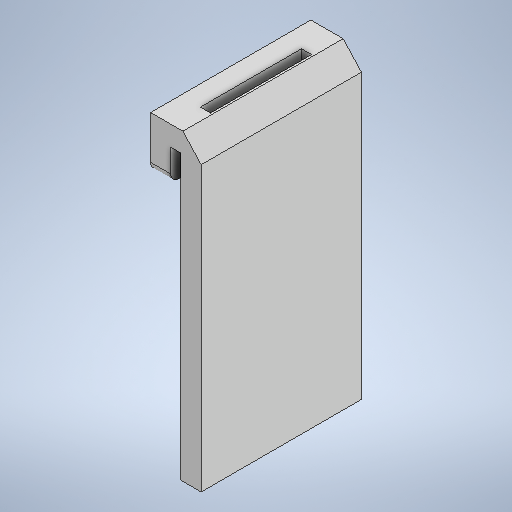
# Autodesk Inventor part: Glass Slide Gripper
Saved by Autodesk Inventor 2025 (Build 290162000, 162)
## iProperties
Created: 2025-04-07
Part Number: Glass Slide Gripper
Material: Generic
Document SubType Name: Modeling
Designer: Caleb Fangmeier
Density: 1 g/cm^3
Appearance: Default
Author: Caleb Fangmeier
Autodesk Inventor part; units mm, degrees
ref_plane "YZ Plane" through (0, 0, 0) normal (1, 0, 0) x (0, 1, 0)
ref_plane "XZ Plane" through (0, 0, 0) normal (0, 1, 0) x (-1, 0, 0)
ref_plane "XY Plane" through (0, 0, 0) normal (0, 0, 1) x (1, 0, 0)
sketch "Sketch1" plane through (0, 0, 0) normal (0, 1, 0) x (-1, 0, 0)
  line L0 (-1.27, -12.7) -> (1.27, -12.7)
  line L1 (1.27, -12.7) -> (1.27, 12.7)
  line L2 (1.27, 12.7) -> (-1.27, 12.7)
  line L3 (-1.27, 12.7) -> (-1.27, -12.7)
  line L4 (-1.27, -12.7) -> (1.27, 12.7) construction
  line L5 (1.27, -12.7) -> (-1.27, 12.7) construction
  line L6 (-6.35, -20.1281) -> (6.35, -20.1281)
  line L7 (6.35, -20.1281) -> (6.35, 20.1281)
  line L8 (6.35, 20.1281) -> (-6.35, 20.1281)
  line L9 (-6.35, 20.1281) -> (-6.35, -20.1281)
  line L10 (-6.35, -20.1281) -> (6.35, 20.1281) construction
  line L11 (6.35, -20.1281) -> (-6.35, 20.1281) construction
  point P0 (0, 0)
  dimension "d0" = 2.54
  dimension "d1" = 25.4
  dimension "d2" = 12.7
  constraints: 24 end point, 4 midpoint, 4 parallel, 2 horizontal, 2 perpendicular
  measures "d0" distance of L1.end L2.end
  measures "d1" distance of L0.end L1.end
  measures "d2" distance of L7.end L8.end
extrude "Extrusion1" add sketch "Sketch1" along normal blind 76.2
sketch "Sketch2" plane through (-6.35, 0, 20.1281) normal (0, 0, 1) x (1, 0, 0)
  line L0 (5.08, 0) -> (5.08, 76.2) projected
  line L1 (7.62, 0) -> (7.62, 76.2) projected
  line L2 (0, 0) -> (12.7, 0) projected
  line L3 (0, 76.2) -> (12.7, 76.2) projected
  line L4 (5.08, 0) -> (5.08, 76.2) projected
  line L5 (5.08, 71.2) -> (7.62, 71.2)
  line L6 (8.12, 76.2) -> (12.7, 71.2)
  line L7 (12.7, 0) -> (12.7, 76.2) projected
  point P0 (6.35, 0)
  dimension "d5" = 5
  dimension "d6" = 0.5
  dimension "d7" = 5
  constraints: 4 end point, 4 point on line, 1 perpendicular
  measures "d5" distance between parallel lines of L5 L3
  measures "d6" distance of L1.end L6.start
  measures "d7" distance of L3.end L6.end
extrude "Extrusion2" cut sketch "Sketch2" against normal through all contours L0 L5 L1 L2 | L6 L3 L7
sketch "Sketch3" plane through (-6.35, 0, -20.1281) normal (-1, 0, 0) x (0, 0, 1)
  line L0 (40.2562, 0) -> (40.2562, 71.2) projected
  arc A0 (40.2562, 63.5) -> (27.5562, 50.8) centre (40.2562, 50.8) ccw
  line L1 (27.5562, 50.8) -> (27.5562, 19.05)
  line L2 (0, 76.2) -> (40.2562, 76.2) projected
  arc A1 (12.7, 19.05) -> (27.5562, 19.05) centre (20.1281, 19.05) ccw
  line L3 (0, 0) -> (0, 76.2) projected
  arc A2 (12.7, 50.8) -> (0, 63.5) centre (0, 50.8) ccw
  line L4 (12.7, 19.05) -> (12.7, 50.8)
  line L5 (0, 0) -> (40.2562, 0) projected
  point P0 (20.1281, 0)
  point P1 (20.1281, 0)
  dimension "d10" = 12.7
  dimension "d11" = 25.4
  dimension "d13" = 19.05
  constraints: 6 point on circle, 4 end point, 4 horizontal alignment, 3 centre point, 3 point on line, 2 tangent, 2 vertical, 1 midpoint, 1 vertical alignment
  measures "d10" distance of A0.centre L1.start
  measures "d11" distance from line of L2 A0.centre
  measures "d13" distance of point (20.128, 0) A1.centre
extrude "Extrusion3" cut sketch "Sketch3" against normal up to surface (5.08 mm away)
fillet "Fillet1" radius 2 2 edges at (-3.81, 63.5, 20.1281) (-3.81, 63.5, -20.1281)
body "Solid1"
